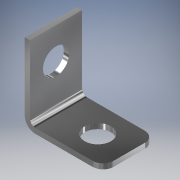
# Autodesk Inventor part: element_clip
Saved by Autodesk Inventor 2018.1 (Build 221171000, 171)
## iProperties
Created: 2017-10-22
Part Number: element_clip
Material: アルミニウム 6061
Document SubType Name: Sheet Metal
Designer: ku_sk
Density: 2.7 g/cm^3
Sheet Metal Rule: Default_mm
Appearance: アルミニウム - フラット
Author: ku_sk
Autodesk Inventor part; units mm, degrees
ref_plane "YZ Plane" through (0, 0, 0) normal (1, 0, 0) x (0, 1, 0)
ref_plane "XZ Plane" through (0, 0, 0) normal (0, 1, 0) x (-1, 0, 0)
ref_plane "XY Plane" through (0, 0, 0) normal (0, 0, 1) x (1, 0, 0)
sketch "スケッチ9" plane through (0, 0, 0) normal (0, 1, 0) x (-1, 0, 0)
  line L0 (5, 7.5) -> (-5, 7.5)
  line L1 (-5, 7.5) -> (-5, -7.5)
  line L2 (-5, -7.5) -> (5, -7.5)
  line L3 (5, -7.5) -> (5, 7.5)
  line L4 (7, 0) -> (-7, 0)
  line L5 (0, -10.5) -> (0, 10.5)
  point P0 (0, 0)
  point P1 (5, 0)
  point P2 (0, 7.5)
  dimension "d53" = 15
  dimension "d54" = 10
  measures "d53" distance of L2.end L0.start
  measures "d54" distance of L0.start L0.end
extrude "プレート7" add sketch "スケッチ9" along normal blind 1
sketch "スケッチ10" plane through (-5, 0, -6.5) normal (0, 0, -1) x (-1, 0, 0)
  line L0 (-10, 0) -> (0, 0)
  line L1 (0, 0) -> (0, 15)
  line L2 (0, 15) -> (-10, 15)
  line L3 (-10, 15) -> (-10, 0)
  constraints: 6 end point, 1 horizontal, 1 perpendicular, 1 vertical
edge flange "フランジ5" height 15 angle 90 thickness 1 bend radius 1 thickness toward (0, 0, -1) relief straight relief width 1 relief depth 0.5 edges at (0, 1, -7.5) wall of the first edge with corners at (5, 0, -6.5) (-5, 0, -6.5) (-5, 15, -6.5) (5, 15, -6.5)
bend "曲げ5"
corner "コーナー5"
sketch "スケッチ11" plane through (-5, 15, -6.5) normal (0, 0, 1) x (1, 0, 0)
  circle A0 centre (5, -6) radius 2.5
  line L0 (10, 0) -> (0, 0) projected
  line L1 (0, 0) -> (0, -13) projected
  point P0 (5, -15)
  dimension "d66" = 5
  dimension "d67" = 6
  dimension "d76" = 5
  constraints: 1 centre point
  measures "d66" diameter of A0
  measures "d67" distance from line of L0 A0.centre
  measures "d76" distance from line of L1 A0.centre
sketch "スケッチ12" plane through (0, 1, 0) normal (0, 1, 0) x (1, 0, 0)
  circle A0 centre (0, -1.5) radius 2.5
  line L0 (5, -7.5) -> (-5, -7.5) projected
  line L1 (-5, -7.5) -> (-5, 5.5) projected
  line L2 (0, 11.6) -> (0, -13.6) projected
  point P0 (0, 0)
  dimension "d69" = 6
  dimension "d71" = 5
  constraints: 1 centre point, 1 point on line
  measures "d69" distance from line of L0 A0.centre
  measures "d71" diameter of A0
extrude "押し出し3" cut sketch "スケッチ12" against normal up to next
extrude "押し出し4" cut sketch "スケッチ11" against normal up to next
fillet "フィレット2" radius 2 2 edges at (5, 0.5, 7.5) (-5, 0.5, 7.5)
equation "\"d55\" = Thickness"
equation "\"d56\" = BendReliefWidth"
equation "\"d57\" = BendReliefDepth"
equation "\"d58\" = MinimumRemnant"
equation "\"d59\" = TransitionRadius"
equation "\"d62\" = BendRadius"
equation "\"d63\" = CornerReliefSize"
equation "\"d64\" = GapSize"
equation "\"d65\" = JacobiRadiusSize"
equation "\"BendRadius\" = Thickness"
equation "\"BendReliefWidth\" = Thickness"
equation "\"BendReliefDepth\" = 0.5 * Thickness"
equation "\"CornerReliefSize\" = 4 * Thickness"
equation "\"MinimumRemnant\" = 2 * Thickness"
equation "\"TransitionRadius\" = BendRadius"
equation "\"JacobiRadiusSize\" = BendRadius"
equation "\"GapSize\" = Thickness"
equation "\"Thickness\" = 1"
